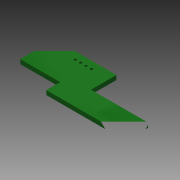
# Autodesk Inventor part: MezzanineBoard
Saved by Autodesk Inventor 2014 (Build 180170000, 170)
## iProperties
Created: 2015-11-05
Part Number: MezzanineBoard
Material: Generic
Document SubType Name: Modeling
Designer: Owner
Density: 1 g/cm^3
Appearance: Smooth - Dark Forest Green
Author: Owner
Autodesk Inventor part; units mm, degrees
ref_plane "YZ Plane" through (0, 0, 0) normal (1, 0, 0) x (0, 1, 0)
ref_plane "XZ Plane" through (0, 0, 0) normal (0, 1, 0) x (-1, 0, 0)
ref_plane "XY Plane" through (0, 0, 0) normal (0, 0, 1) x (1, 0, 0)
sketch "Sketch1" plane through (0, 0, 0) normal (0, 1, 0) x (-1, 0, 0)
  line L0 (-14.7409, 8.9608) -> (29.2011, 8.9608)
  line L1 (29.2011, 8.9608) -> (29.2011, -8.8192)
  line L2 (29.2011, -8.8192) -> (-14.7409, -8.8192)
  line L3 (-14.7409, -8.8192) -> (-14.7409, 8.9608)
  line L4 (-14.7409, 8.9608) -> (14.4691, 8.9608)
  line L5 (14.4691, 8.9608) -> (14.4691, 3.8808)
  line L6 (6.3411, 0.5788) -> (-14.7409, 0.5788)
  line L7 (-14.7409, 0.5788) -> (-14.7409, 8.9608)
  line L8 (29.2011, -8.8192) -> (6.3411, -8.8192)
  line L9 (6.3411, -8.8192) -> (6.3411, 0.5788)
  line L10 (14.4691, 3.8808) -> (29.2011, 3.8808)
  line L11 (29.2011, 3.8808) -> (29.2011, -8.8192)
  point P0 (0, 0)
  dimension "d0" = 43.942
  dimension "d1" = 17.78
  dimension "d2" = 21.082
  dimension "d3" = 14.732
  dimension "d4" = 9.398
  dimension "d5" = 5.08
  constraints: 24 end point, 6 parallel, 3 horizontal, 3 perpendicular
  measures "d0" distance of L0.start L0.end
  measures "d1" distance of L2.end L0.start
  measures "d2" distance of L6.start L6.end
  measures "d3" distance of L5.end L10.end
  measures "d4" distance of L8.end L6.start
  measures "d5" distance of L4.end L5.end
extrude "Extrusion1" add sketch "Sketch1" along normal blind 1.6 contours L0 L5 L10 L1 L2 L9 L6 L3
sketch "Sketch2" plane through (0, 1.6, 0) normal (0, 1, 0) x (1, 0, 0)
  line L0 (-6.3411, -0.5788) -> (-6.3411, 8.8192) projected
  line L1 (-6.3411, 8.8192) -> (-29.2011, 8.8192) projected
  line L2 (-14.4691, -8.9608) -> (14.7409, -8.9608) projected
  circle A0 centre (-12.8689, 6.3808) radius 0.45
  line L3 (-18.8689, 6.3808) -> (-12.8689, 6.3808) construction
  circle A1 centre (-14.8689, 6.3808) radius 0.45
  circle A2 centre (-16.8689, 6.3808) radius 0.45
  circle A3 centre (-18.8689, 6.3808) radius 0.45
  point P0 (0, 0)
  dimension "d9" = 6.5278
  dimension "d15" = 0.9
  dimension "d16" = 2.4384
  dimension "d19" = 0.9
  dimension "d20" = 0.9
  dimension "d21" = 0.9
  dimension "d22" = 2
  dimension "d23" = 2
  dimension "d24" = 2
  constraints: 4 centre point, 3 point on line, 2 end point, 1 parallel
  measures "d9" distance from line of L0 L3.end
  measures "d15" diameter of A0
  measures "d16" distance from line of L1 L3.end
  measures "d19" diameter of A1
  measures "d20" diameter of A2
  measures "d21" diameter of A3
  measures "d22" distance of A1.centre L3.end
  measures "d23" distance of A1.centre A2.centre
  measures "d24" distance of A3.centre A2.centre
extrude "Extrusion2" cut sketch "Sketch2" against normal up to next
body "Solid1"
